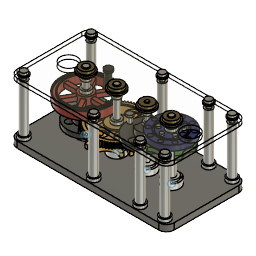
DualStageGenevaIndexingMechanism_2_5D_AI_Model (Autodesk Fusion 360 design; units mm, degrees)
part number: 2026-08-16-05-34-55-239
part number: 2026-08-16-05-35-11-169
part number: 2026-08-16-05-35-42-913
part number: 2026-08-16-05-35-42-976
part number: 2026-08-16-05-35-43-045
part number: 2026-08-16-05-35-43-120
part number: 2026-08-16-05-35-43-201
part number: 2026-08-16-05-36-34-609
part number: 2026-08-16-05-36-34-765
part number: 2026-08-16-05-36-34-899
part number: 2026-08-16-05-36-35-022
part number: 2026-08-16-05-37-12-410
part number: 2026-08-16-05-37-12-675
part number: 2026-08-16-05-39-24-332
part number: 2026-08-16-05-39-24-566
part number: 2026-08-16-05-40-07-479
part number: 2026-08-16-05-41-21-230
part number: 2026-08-16-05-43-01-261
part number: 2026-08-16-05-43-01-779
part number: 2026-08-16-05-43-02-149
part number: 2026-08-16-05-44-14-801
part number: 2026-08-16-05-44-15-447
part number: 2026-08-16-05-45-26-077
part number: 2026-08-16-05-45-26-591
part number: 2026-08-16-05-45-26-921
part number: 2026-08-16-05-45-27-444
Autodesk Fusion 360 part; units mm, degrees
note: some values were not read from the file. Chosen so that the rebuilt part matches the saved one: which bodies a step acts on. Set by a fixed rule: which sketch regions a step uses.
(part 1 of 6)
sketch "スケッチ1" plane through (0, 0, 0) normal (0, 0, 1) x (1, 0, 0) in component "Lower_Base_Plate"
  line L0 (-290, -125) -> (200, -125)
  line L1 (200, -125) -> (200, 125)
  line L2 (200, 125) -> (-290, 125)
  line L3 (-290, 125) -> (-290, -125)
extrude "押し出し1" add sketch "スケッチ1" along normal blind 20 from surface at -20 makes body 1 in component "Lower_Base_Plate"
fillet "フィレット1" radius 24 4 edges at (-290, 125, -10) (200, 125, -10) (200, -125, -10) (-290, -125, -10) on bodies 1 in component "Lower_Base_Plate"
sketch "スケッチ1 (2)" plane through (0, 0, 0) normal (0, 0, 1) x (1, 0, 0) in component "Bearing_Housing_A"
  circle A0 centre (-176, 0) radius 26
extrude "押し出し1'" add sketch "スケッチ1 (2)" along normal blind 18 separate body makes body 2 in component "Bearing_Housing_A"
sketch "スケッチ2" plane through (0, 0, 0) normal (0, 0, 1) x (1, 0, 0) in component "Bearing_Housing_A"
  circle A0 centre (-176, 0) radius 20
extrude "押し出し2" add sketch "スケッチ2" along normal blind 6 from surface at 18 bodies 2 in component "Bearing_Housing_A"
sketch "スケッチ3" plane through (0, 0, 0) normal (0, 0, 1) x (1, 0, 0) in component "Bearing_Housing_A"
  circle A0 centre (-176, 0) radius 10
  circle A1 centre (-160.0901, 15.9099) radius 3
  circle A2 centre (-191.9099, 15.9099) radius 3
  circle A3 centre (-191.9099, -15.9099) radius 3
  circle A4 centre (-160.0901, -15.9099) radius 3
extrude "押し出し3" cut sketch "スケッチ3" along normal blind 40 from surface at -5 bodies 2 in component "Bearing_Housing_A"
sketch "スケッチ1 (3)" plane through (0, 0, 0) normal (0, 0, 1) x (1, 0, 0) in component "Bearing_Housing_B"
  circle A0 centre (-80, 0) radius 26
extrude "押し出し1''" add sketch "スケッチ1 (3)" along normal blind 18 separate body makes body 3 in component "Bearing_Housing_B"
sketch "スケッチ2 (2)" plane through (0, 0, 0) normal (0, 0, 1) x (1, 0, 0) in component "Bearing_Housing_B"
  circle A0 centre (-80, 0) radius 20
extrude "押し出し2'" add sketch "スケッチ2 (2)" along normal blind 6 from surface at 18 bodies 3 in component "Bearing_Housing_B"
sketch "スケッチ3 (2)" plane through (0, 0, 0) normal (0, 0, 1) x (1, 0, 0) in component "Bearing_Housing_B"
  circle A0 centre (-80, 0) radius 9
  circle A1 centre (-64.0901, 15.9099) radius 3
  circle A2 centre (-95.9099, 15.9099) radius 3
  circle A3 centre (-95.9099, -15.9099) radius 3
  circle A4 centre (-64.0901, -15.9099) radius 3
extrude "押し出し3'" cut sketch "スケッチ3 (2)" along normal blind 40 from surface at -5 bodies 3 in component "Bearing_Housing_B"
sketch "スケッチ1 (4)" plane through (0, 0, 0) normal (0, 0, 1) x (1, 0, 0) in component "Bearing_Housing_C"
  circle A0 centre (14.5, 0) radius 26
extrude "押し出し1'''" add sketch "スケッチ1 (4)" along normal blind 18 separate body makes body 4 in component "Bearing_Housing_C"
sketch "スケッチ2 (3)" plane through (0, 0, 0) normal (0, 0, 1) x (1, 0, 0) in component "Bearing_Housing_C"
  circle A0 centre (14.5, 0) radius 20
extrude "押し出し2''" add sketch "スケッチ2 (3)" along normal blind 6 from surface at 18 bodies 4 in component "Bearing_Housing_C"
sketch "スケッチ3 (3)" plane through (0, 0, 0) normal (0, 0, 1) x (1, 0, 0) in component "Bearing_Housing_C"
  circle A0 centre (14.5, 0) radius 6
  circle A1 centre (30.4099, 15.9099) radius 3
  circle A2 centre (-1.4099, 15.9099) radius 3
  circle A3 centre (-1.4099, -15.9099) radius 3
  circle A4 centre (30.4099, -15.9099) radius 3
extrude "押し出し3''" cut sketch "スケッチ3 (3)" along normal blind 40 from surface at -5 bodies 4 in component "Bearing_Housing_C"
sketch "スケッチ1 (5)" plane through (0, 0, 0) normal (0, 0, 1) x (1, 0, 0) in component "Bearing_Housing_D"
  circle A0 centre (90.5, 0) radius 26
extrude "押し出し1''''" add sketch "スケッチ1 (5)" along normal blind 18 separate body makes body 5 in component "Bearing_Housing_D"
sketch "スケッチ2 (4)" plane through (0, 0, 0) normal (0, 0, 1) x (1, 0, 0) in component "Bearing_Housing_D"
  circle A0 centre (90.5, 0) radius 20
extrude "押し出し2'''" add sketch "スケッチ2 (4)" along normal blind 6 from surface at 18 bodies 5 in component "Bearing_Housing_D"
sketch "スケッチ3 (4)" plane through (0, 0, 0) normal (0, 0, 1) x (1, 0, 0) in component "Bearing_Housing_D"
  circle A0 centre (90.5, 0) radius 9
  circle A1 centre (106.4099, 15.9099) radius 3
  circle A2 centre (74.5901, 15.9099) radius 3
  circle A3 centre (74.5901, -15.9099) radius 3
  circle A4 centre (106.4099, -15.9099) radius 3
extrude "押し出し3'''" cut sketch "スケッチ3 (4)" along normal blind 40 from surface at -5 bodies 5 in component "Bearing_Housing_D"
sketch "スケッチ1 (6)" plane through (0, 0, 0) normal (0, 0, 1) x (1, 0, 0) in component "Standoff_Posts"
  circle A0 centre (-265, 105) radius 12
  circle A1 centre (-265, -105) radius 12
  circle A2 centre (-45, 107) radius 12
  circle A3 centre (-45, -107) radius 12
  circle A4 centre (100, 107) radius 12
  circle A5 centre (100, -107) radius 12
  circle A6 centre (175, 105) radius 12
  circle A7 centre (175, -105) radius 12
extrude "押し出し1'''''" add sketch "スケッチ1 (6)" along normal blind 158 separate body makes body 6 at (186.9404, 103.8052, 105.3333) makes body 7 at (111.9404, 105.8052, 105.3333) makes body 8 at (-33.0596, -108.1948, 105.3333) makes body 9 at (-270.4745, -115.6785, 52.6667) makes body 10 at (-33.0596, 105.8052, 105.3333) makes body 11 at (-270.4745, 94.3215, 52.6667) makes body 12 at (111.9404, -108.1948, 105.3333) makes body 13 at (186.9404, -106.1948, 105.3333) in component "Standoff_Posts"
sketch "スケッチ2 (5)" plane through (0, 0, 0) normal (0, 0, 1) x (1, 0, 0) in component "Standoff_Posts"
  circle A0 centre (-265, 105) radius 16
  circle A1 centre (-265, -105) radius 16
  circle A2 centre (-45, 107) radius 16
  circle A3 centre (-45, -107) radius 16
  circle A4 centre (100, 107) radius 16
  circle A5 centre (100, -107) radius 16
  circle A6 centre (175, 105) radius 16
  circle A7 centre (175, -105) radius 16
extrude "押し出し2''''" add sketch "スケッチ2 (5)" along normal blind 10 bodies 6 7 8 9 10 11 12 13 in component "Standoff_Posts"
sketch "スケッチ3 (5)" plane through (0, 0, 0) normal (0, 0, 1) x (1, 0, 0) in component "Standoff_Posts"
  circle A0 centre (-265, 105) radius 6
  circle A1 centre (-265, -105) radius 6
  circle A2 centre (-45, 107) radius 6
  circle A3 centre (-45, -107) radius 6
  circle A4 centre (100, 107) radius 6
  circle A5 centre (100, -107) radius 6
  circle A6 centre (175, 105) radius 6
  circle A7 centre (175, -105) radius 6
extrude "押し出し3''''" cut sketch "スケッチ3 (5)" along normal blind 20 from surface at 140 bodies 6 7 8 9 10 11 12 13 in component "Standoff_Posts"
sketch "スケッチ1 (7)" plane through (0, 0, 0) normal (0, 0, 1) x (1, 0, 0) in component "Input_Shaft"
  circle A0 centre (-176, 0) radius 9
extrude "押し出し1''''''" add sketch "スケッチ1 (7)" along normal blind 186 separate body makes body 14 in component "Input_Shaft"
sketch "スケッチ2 (6)" plane through (0, 0, 0) normal (0, 0, 1) x (1, 0, 0) in component "Input_Shaft"
  circle A0 centre (-176, 0) radius 14
extrude "押し出し2'''''" add sketch "スケッチ2 (6)" along normal blind 4 from surface at 24 bodies 14 in component "Input_Shaft"
sketch "スケッチ3 (6)" plane through (0, 0, 0) normal (0, 0, 1) x (1, 0, 0) in component "Input_Shaft"
  circle A0 centre (-176, 0) radius 10
extrude "押し出し3'''''" add sketch "スケッチ3 (6)" along normal blind 20 from surface at 62 bodies 14 in component "Input_Shaft"
sketch "スケッチ4" plane through (0, 0, 0) normal (0, 0, 1) x (1, 0, 0) in component "Input_Shaft"
  circle A0 centre (-176, 0) radius 11
extrude "押し出し4" add sketch "スケッチ4" along normal blind 10 from surface at 82 bodies 14 in component "Input_Shaft"
sketch "スケッチ5" plane through (0, 0, 0) normal (0, 0, 1) x (1, 0, 0) in component "Input_Shaft"
  circle A0 centre (-176, 0) radius 15
extrude "押し出し5" add sketch "スケッチ5" along normal blind 10 from surface at 117 bodies 14 in component "Input_Shaft"
sketch "スケッチ6" plane through (0, 0, 0) normal (0, 0, 1) x (1, 0, 0) in component "Input_Shaft"
  circle A0 centre (-176, 0) radius 13
extrude "押し出し6" add sketch "スケッチ6" along normal blind 8 from surface at 150 bodies 14 in component "Input_Shaft"
sketch "スケッチ7" plane through (0, 0, 0) normal (0, 0, 1) x (1, 0, 0) in component "Input_Shaft"
  circle A0 centre (-176, 0) radius 10.8
sketch "スケッチ1 (8)" plane through (0, 0, 0) normal (0, 0, 1) x (1, 0, 0) in component "Stage1_Shaft"
  circle A0 centre (-80, 0) radius 8
extrude "押し出し1'''''''" add sketch "スケッチ1 (8)" along normal blind 186 separate body makes body 15 in component "Stage1_Shaft"
sketch "スケッチ2 (7)" plane through (0, 0, 0) normal (0, 0, 1) x (1, 0, 0) in component "Stage1_Shaft"
  circle A0 centre (-80, 0) radius 14
extrude "押し出し2''''''" add sketch "スケッチ2 (7)" along normal blind 20 from surface at 24 bodies 15 in component "Stage1_Shaft"
sketch "スケッチ3 (7)" plane through (0, 0, 0) normal (0, 0, 1) x (1, 0, 0) in component "Stage1_Shaft"
  circle A0 centre (-80, 0) radius 14
extrude "押し出し3''''''" add sketch "スケッチ3 (7)" along normal blind 6 from surface at 60 bodies 15 in component "Stage1_Shaft"
sketch "スケッチ4 (2)" plane through (0, 0, 0) normal (0, 0, 1) x (1, 0, 0) in component "Stage1_Shaft"
  circle A0 centre (-80, 0) radius 15
extrude "押し出し4'" add sketch "スケッチ4 (2)" along normal blind 10 from surface at 82 bodies 15 in component "Stage1_Shaft"
sketch "スケッチ5 (2)" plane through (0, 0, 0) normal (0, 0, 1) x (1, 0, 0) in component "Stage1_Shaft"
  circle A0 centre (-80, 0) radius 12
extrude "押し出し5'" add sketch "スケッチ5 (2)" along normal blind 8 from surface at 150 bodies 15 in component "Stage1_Shaft"
sketch "スケッチ6 (2)" plane through (0, 0, 0) normal (0, 0, 1) x (1, 0, 0) in component "Stage1_Shaft"
  circle A0 centre (-80, 0) radius 9.8
sketch "スケッチ1 (9)" plane through (0, 0, 0) normal (0, 0, 1) x (1, 0, 0) in component "Stage2_Driver_Shaft"
  circle A0 centre (14.5, 0) radius 5
extrude "押し出し1''''''''" add sketch "スケッチ1 (9)" along normal blind 186 separate body makes body 16 in component "Stage2_Driver_Shaft"
sketch "スケッチ2 (8)" plane through (0, 0, 0) normal (0, 0, 1) x (1, 0, 0) in component "Stage2_Driver_Shaft"
  circle A0 centre (14.5, 0) radius 7
extrude "押し出し2'''''''" add sketch "スケッチ2 (8)" along normal blind 42 from surface at 24 bodies 16 in component "Stage2_Driver_Shaft"
sketch "スケッチ3 (8)" plane through (0, 0, 0) normal (0, 0, 1) x (1, 0, 0) in component "Stage2_Driver_Shaft"
  circle A0 centre (14.5, 0) radius 11
extrude "押し出し3'''''''" add sketch "スケッチ3 (8)" along normal blind 10 from surface at 122 bodies 16 in component "Stage2_Driver_Shaft"
sketch "スケッチ4 (3)" plane through (0, 0, 0) normal (0, 0, 1) x (1, 0, 0) in component "Stage2_Driver_Shaft"
  circle A0 centre (14.5, 0) radius 9
extrude "押し出し4''" add sketch "スケッチ4 (3)" along normal blind 8 from surface at 150 bodies 16 in component "Stage2_Driver_Shaft"
sketch "スケッチ5 (3)" plane through (0, 0, 0) normal (0, 0, 1) x (1, 0, 0) in component "Stage2_Driver_Shaft"
  circle A0 centre (14.5, 0) radius 6.8
sketch "スケッチ1 (10)" plane through (0, 0, 0) normal (0, 0, 1) x (1, 0, 0) in component "Output_Shaft"
  circle A0 centre (90.5, 0) radius 8
extrude "押し出し1'''''''''" add sketch "スケッチ1 (10)" along normal blind 186 separate body makes body 17 in component "Output_Shaft"
sketch "スケッチ2 (9)" plane through (0, 0, 0) normal (0, 0, 1) x (1, 0, 0) in component "Output_Shaft"
  circle A0 centre (90.5, 0) radius 12
extrude "押し出し2''''''''" add sketch "スケッチ2 (9)" along normal blind 76 from surface at 24 bodies 17 in component "Output_Shaft"
sketch "スケッチ3 (9)" plane through (0, 0, 0) normal (0, 0, 1) x (1, 0, 0) in component "Output_Shaft"
  circle A0 centre (90.5, 0) radius 15
extrude "押し出し3''''''''" add sketch "スケッチ3 (9)" along normal blind 10 from surface at 148 bodies 17 in component "Output_Shaft"
sketch "スケッチ4 (4)" plane through (0, 0, 0) normal (0, 0, 1) x (1, 0, 0) in component "Output_Shaft"
  circle A0 centre (90.5, 0) radius 11.15
sketch "スケッチ1 (11)" plane through (0, 0, 0) normal (0, 0, 1) x (1, 0, 0) in component "Input_Handwheel"
  circle A0 centre (-176, 0) radius 78
  circle A1 centre (-176, 0) radius 64
extrude "押し出し1''''''''''" add sketch "スケッチ1 (11)" along normal blind 25 from surface at 92 separate body makes body 18 in component "Input_Handwheel"
sketch "スケッチ2 (10)" plane through (0, 0, 0) normal (0, 0, 1) x (1, 0, 0) in component "Input_Handwheel"
  circle A0 centre (-176, 0) radius 22
  circle A1 centre (-176, 0) radius 9
extrude "押し出し2'''''''''" add sketch "スケッチ2 (10)" along normal blind 25 from surface at 92 bodies 18 makes body 19 in component "Input_Handwheel"
sketch "スケッチ3 (10)" plane through (0, 0, 0) normal (0, 0, 1) x (1, 0, 0) in component "Input_Handwheel"
  line L0 (-160, 6) -> (-110, 6)
  line L1 (-110, 6) -> (-110, -6)
  line L2 (-110, -6) -> (-160, -6)
  line L3 (-160, -6) -> (-160, 6)
  line L4 (-173.1962, 16.8564) -> (-148.1962, 60.1577)
  line L5 (-148.1962, 60.1577) -> (-137.8038, 54.1577)
  line L6 (-137.8038, 54.1577) -> (-162.8038, 10.8564)
  line L7 (-162.8038, 10.8564) -> (-173.1962, 16.8564)
  line L8 (-189.1962, 10.8564) -> (-214.1962, 54.1577)
  line L9 (-214.1962, 54.1577) -> (-203.8038, 60.1577)
  line L10 (-203.8038, 60.1577) -> (-178.8038, 16.8564)
  line L11 (-178.8038, 16.8564) -> (-189.1962, 10.8564)
  line L12 (-192, -6) -> (-242, -6)
  line L13 (-242, -6) -> (-242, 6)
  line L14 (-242, 6) -> (-192, 6)
  line L15 (-192, 6) -> (-192, -6)
  line L16 (-178.8038, -16.8564) -> (-203.8038, -60.1577)
  line L17 (-203.8038, -60.1577) -> (-214.1962, -54.1577)
  line L18 (-214.1962, -54.1577) -> (-189.1962, -10.8564)
  line L19 (-189.1962, -10.8564) -> (-178.8038, -16.8564)
  line L20 (-162.8038, -10.8564) -> (-137.8038, -54.1577)
  line L21 (-137.8038, -54.1577) -> (-148.1962, -60.1577)
  line L22 (-148.1962, -60.1577) -> (-173.1962, -16.8564)
  line L23 (-173.1962, -16.8564) -> (-162.8038, -10.8564)
extrude "押し出し3'''''''''" add sketch "スケッチ3 (10)" along normal blind 13 from surface at 98 bodies 18 in component "Input_Handwheel"
sketch "スケッチ4 (5)" plane through (0, 0, 0) normal (0, 0, 1) x (1, 0, 0) in component "Input_Handwheel"
  circle A0 centre (-176, 0) radius 75
  circle A1 centre (-176, 0) radius 67
extrude "押し出し4'''" cut sketch "スケッチ4 (5)" along normal blind 5 from surface at 113 bodies 18 in component "Input_Handwheel"
sketch "スケッチ1 (12)" plane through (0, 0, 0) normal (0, 0, 1) x (1, 0, 0) in component "Input_Crank_Handle"
  circle A0 centre (-176, 70) radius 9
extrude "押し出し1'''''''''''" add sketch "スケッチ1 (12)" along normal blind 32 from surface at 106 separate body makes body 20 in component "Input_Crank_Handle"
sketch "スケッチ2 (11)" plane through (0, 0, 0) normal (0, 0, 1) x (1, 0, 0) in component "Input_Crank_Handle"
  circle A0 centre (-176, 70) radius 12
extrude "押し出し2''''''''''" add sketch "スケッチ2 (11)" along normal blind 6 from surface at 138 bodies 20 in component "Input_Crank_Handle"
sketch "スケッチ5 (4)" plane through (0, 0, 0) normal (0, 0, 1) x (1, 0, 0) in component "Input_Handwheel"
  circle A0 centre (-176, 70) radius 9.4
extrude "押し出し5''" cut sketch "スケッチ5 (4)" along normal blind 36 from surface at 86 bodies 18 in component "Input_Handwheel"
sketch "スケッチ3 (11)" plane through (0, 0, 0) normal (0, 0, 1) x (1, 0, 0) in component "Input_Crank_Handle"
  circle A0 centre (-176, 70) radius 9
extrude "押し出し3''''''''''" add sketch "スケッチ3 (11)" along normal blind 14 from surface at 92 bodies 20 in component "Input_Crank_Handle"
sketch "スケッチ4 (6)" plane through (0, 0, 0) normal (0, 0, 1) x (1, 0, 0) in component "Input_Crank_Handle"
  circle A0 centre (-176, 70) radius 13
extrude "押し出し4''''" add sketch "スケッチ4 (6)" along normal blind 8 from surface at 84 bodies 20 in component "Input_Crank_Handle"
combine "結合1" operation add target body 18 tool bodies 19 in component "Input_Handwheel"
sketch "スケッチ1 (13)" plane through (0, 0, 0) normal (0, 0, 1) x (1, 0, 0) in component "Stage1_Driver_Disc"
  circle A0 centre (-176, 0) radius 58
extrude "押し出し1''''''''''''" add sketch "スケッチ1 (13)" along normal blind 14 from surface at 28 separate body makes body 21 in component "Stage1_Driver_Disc"
sketch "スケッチ2 (12)" plane through (0, 0, 0) normal (0, 0, 1) x (1, 0, 0) in component "Stage1_Driver_Disc"
  circle A0 centre (-176, 0) radius 16
extrude "押し出し2'''''''''''" add sketch "スケッチ2 (12)" along normal blind 34 from surface at 28 bodies 21 in component "Stage1_Driver_Disc"
sketch "スケッチ3 (12)" plane through (0, 0, 0) normal (0, 0, 1) x (1, 0, 0) in component "Stage1_Driver_Disc"
  circle A0 centre (-176, 0) radius 32
  circle A1 centre (-128, 83.1384) radius 86
extrude "押し出し3'''''''''''" add sketch "スケッチ3 (12)" along normal blind 20 from surface at 42 contours A0 A1 picked at (-177.9353, -3.352) bodies 21 in component "Stage1_Driver_Disc"
sketch "スケッチ4 (7)" plane through (0, 0, 0) normal (0, 0, 1) x (1, 0, 0) in component "Stage1_Driver_Disc"
  circle A0 centre (-208.909, 19) radius 11
  circle A1 centre (-195, -32.909) radius 11
  circle A2 centre (-143.091, -19) radius 11
extrude "押し出し4'''''" cut sketch "スケッチ4 (7)" along normal blind 14 from surface at 28 bodies 21 in component "Stage1_Driver_Disc"
sketch "スケッチ5 (5)" plane through (0, 0, 0) normal (0, 0, 1) x (1, 0, 0) in component "Stage1_Driver_Disc"
  circle A0 centre (-176, 0) radius 9
extrude "押し出し5'''" cut sketch "スケッチ5 (5)" along normal blind 42 from surface at 24 bodies 21 in component "Stage1_Driver_Disc"
sketch "スケッチ1 (14)" plane through (0, 0, 0) normal (0, 0, 1) x (1, 0, 0) in component "Stage1_Drive_Pin"
  circle A0 centre (-152, 41.5692) radius 6
extrude "押し出し1'''''''''''''" add sketch "スケッチ1 (14)" along normal blind 22 from surface at 42 separate body makes body 22 in component "Stage1_Drive_Pin"
sketch "スケッチ2 (13)" plane through (0, 0, 0) normal (0, 0, 1) x (1, 0, 0) in component "Stage1_Drive_Pin"
  circle A0 centre (-152, 41.5692) radius 9.5
extrude "押し出し2''''''''''''" add sketch "スケッチ2 (13)" along normal blind 6 from surface at 58 bodies 22 in component "Stage1_Drive_Pin"
sketch "スケッチ1 (15)" plane through (0, 0, 0) normal (0, 0, 1) x (1, 0, 0) in component "Stage1_Geneva_Wheel_6Slot"
  circle A0 centre (-80, 0) radius 85
extrude "押し出し1''''''''''''''" add sketch "スケッチ1 (15)" along normal blind 12 from surface at 46 separate body makes body 23 in component "Stage1_Geneva_Wheel_6Slot"
sketch "スケッチ2 (14)" plane through (0, 0, 0) normal (0, 0, 1) x (1, 0, 0) in component "Stage1_Geneva_Wheel_6Slot"
  circle A0 centre (-80, 0) radius 22
extrude "押し出し2'''''''''''''" add sketch "スケッチ2 (14)" along normal blind 16 from surface at 44 bodies 23 in component "Stage1_Geneva_Wheel_6Slot"
sketch "スケッチ3 (13)" plane through (0, 0, 0) normal (0, 0, 1) x (1, 0, 0) in component "Stage1_Geneva_Wheel_6Slot"
  line L0 (-124.8192, 18.3708) -> (-163.7904, 40.8708)
  line L1 (-163.7904, 40.8708) -> (-157.2904, 52.1292)
  line L2 (-157.2904, 52.1292) -> (-118.3192, 29.6292)
  arc A0 (-124.8192, 18.3708) -> (-118.3192, 29.6292) centre (-121.5692, 24) ccw
  line L3 (-118.3192, -29.6292) -> (-157.2904, -52.1292)
  line L4 (-157.2904, -52.1292) -> (-163.7904, -40.8708)
  line L5 (-163.7904, -40.8708) -> (-124.8192, -18.3708)
  arc A1 (-118.3192, -29.6292) -> (-124.8192, -18.3708) centre (-121.5692, -24) ccw
  line L6 (-73.5, -48) -> (-73.5, -93)
  line L7 (-73.5, -93) -> (-86.5, -93)
  line L8 (-86.5, -93) -> (-86.5, -48)
  arc A2 (-73.5, -48) -> (-86.5, -48) centre (-80, -48) ccw
  line L9 (-35.1808, -18.3708) -> (3.7904, -40.8708)
  line L10 (3.7904, -40.8708) -> (-2.7096, -52.1292)
  line L11 (-2.7096, -52.1292) -> (-41.6808, -29.6292)
  arc A3 (-35.1808, -18.3708) -> (-41.6808, -29.6292) centre (-38.4308, -24) ccw
  line L12 (-41.6808, 29.6292) -> (-2.7096, 52.1292)
  line L13 (-2.7096, 52.1292) -> (3.7904, 40.8708)
  line L14 (3.7904, 40.8708) -> (-35.1808, 18.3708)
  arc A4 (-41.6808, 29.6292) -> (-35.1808, 18.3708) centre (-38.4308, 24) ccw
  line L15 (-86.5, 48) -> (-86.5, 93)
  line L16 (-86.5, 93) -> (-73.5, 93)
  line L17 (-73.5, 93) -> (-73.5, 48)
  arc A5 (-86.5, 48) -> (-73.5, 48) centre (-80, 48) ccw
extrude "押し出し3''''''''''''" cut sketch "スケッチ3 (13)" along normal blind 20 from surface at 42 bodies 23 in component "Stage1_Geneva_Wheel_6Slot"
sketch "スケッチ4 (8)" plane through (0, 0, 0) normal (0, 0, 1) x (1, 0, 0) in component "Stage1_Geneva_Wheel_6Slot"
  circle A0 centre (-176, 0) radius 32
  circle A1 centre (-128, -83.1384) radius 32
  circle A2 centre (-32, -83.1384) radius 32
  circle A3 centre (16, 0) radius 32
  circle A4 centre (-32, 83.1384) radius 32
  circle A5 centre (-128, 83.1384) radius 32
extrude "押し出し4''''''" cut sketch "スケッチ4 (8)" along normal blind 20 from surface at 42 bodies 23 in component "Stage1_Geneva_Wheel_6Slot"
sketch "スケッチ5 (6)" plane through (0, 0, 0) normal (0, 0, 1) x (1, 0, 0) in component "Stage1_Geneva_Wheel_6Slot"
  circle A0 centre (-122, 0) radius 11
  circle A1 centre (-101, -36.3731) radius 11
  circle A2 centre (-59, -36.3731) radius 11
  circle A3 centre (-38, 0) radius 11
  circle A4 centre (-59, 36.3731) radius 11
  circle A5 centre (-101, 36.3731) radius 11
extrude "押し出し5''''" cut sketch "スケッチ5 (6)" along normal blind 20 from surface at 42 bodies 23 in component "Stage1_Geneva_Wheel_6Slot"
sketch "スケッチ6 (3)" plane through (0, 0, 0) normal (0, 0, 1) x (1, 0, 0) in component "Stage1_Geneva_Wheel_6Slot"
  circle A0 centre (-80, 0) radius 8
extrude "押し出し6'" cut sketch "スケッチ6 (3)" along normal blind 24 from surface at 40 bodies 23 in component "Stage1_Geneva_Wheel_6Slot"
sketch "スケッチ1 (16)" plane through (0, 0, 0) normal (0, 0, 1) x (1, 0, 0) in component "Intermediate_Spur_Gear_72T"
  spline S0 degree 5 poles (3.2013, 2.8471) (3.1556, 2.825) (3.0643, 2.7811) (2.9279, 2.7161) (2.7471, 2.631) (2.5228, 2.5275) (2.3003, 2.4268) (2.0797, 2.329) (1.8609, 2.2341) (1.644, 2.1421) (1.4292, 2.0529) (1.2166, 1.9667) (1.0061, 1.8834) (0.798, 1.8029) (0.5923, 1.7252) (0.389, 1.6503) (0.1883, 1.5783) (-0.0098, 1.5091) (-0.2052, 1.4426) (-0.3978, 1.379) (-0.5873, 1.3182) (-0.7737, 1.2602) (-0.9567, 1.2049) (-1.1363, 1.1524) (-1.3124, 1.1026) (-1.4849, 1.0555) (-1.6201, 1.02) (-1.7199, 0.9945) (-1.7858, 0.9781) (-1.8185, 0.97) knots 0 0 0 0 0 0 0.04 0.08 0.12 0.16 0.2 0.24 0.28 0.32 0.36 0.4 0.44 0.48 0.52 0.56 0.6 0.64 0.68 0.72 0.76 0.8 0.84 0.88 0.92 0.96 1 1 1 1 1 1
  arc A0 (-1.8185, 0.97) -> (3.1328, 4.4152) centre (-0.1573, 3.8631) ccw
  spline S1 degree 5 poles (3.1328, 4.4152) (3.0854, 4.4332) (2.9906, 4.469) (2.8491, 4.5219) (2.6616, 4.5909) (2.4291, 4.6744) (2.1987, 4.7554) (1.9703, 4.8336) (1.7441, 4.9091) (1.52, 4.9818) (1.2983, 5.0519) (1.0789, 5.1193) (0.862, 5.184) (0.6477, 5.246) (0.436, 5.3055) (0.227, 5.3623) (0.0207, 5.4166) (-0.1827, 5.4683) (-0.3831, 5.5174) (-0.5805, 5.564) (-0.7746, 5.6081) (-0.9653, 5.6497) (-1.1525, 5.6888) (-1.336, 5.7254) (-1.5157, 5.7596) (-1.6917, 5.7915) (-1.8295, 5.8151) (-1.9311, 5.8318) (-1.9982, 5.8425) (-2.0315, 5.8477) knots 0 0 0 0 0 0 0.04 0.08 0.12 0.16 0.2 0.24 0.28 0.32 0.36 0.4 0.44 0.48 0.52 0.56 0.6 0.64 0.68 0.72 0.76 0.8 0.84 0.88 0.92 0.96 1 1 1 1 1 1
  arc A1 (2.6366, 10.0878) -> (-2.0315, 5.8477) centre (1.5239, 6.6231) ccw
  spline S2 degree 5 poles (2.6366, 10.0878) (2.5929, 10.0618) (2.5058, 10.0101) (2.3757, 9.9334) (2.2029, 9.8329) (1.9885, 9.7102) (1.7757, 9.5905) (1.5643, 9.4739) (1.3546, 9.3602) (1.1466, 9.2496) (0.9404, 9.1422) (0.7361, 9.0377) (0.5337, 8.9363) (0.3334, 8.838) (0.1352, 8.7427) (-0.0607, 8.6504) (-0.2544, 8.5612) (-0.4457, 8.4749) (-0.6346, 8.3917) (-0.8209, 8.3116) (-1.0044, 8.2345) (-1.185, 8.1604) (-1.3625, 8.0894) (-1.5369, 8.0214) (-1.7079, 7.9565) (-1.8757, 7.8946) (-2.0073, 7.8474) (-2.1045, 7.8133) (-2.1686, 7.7912) (-2.2006, 7.7802) knots 0 0 0 0 0 0 0.04 0.08 0.12 0.16 0.2 0.24 0.28 0.32 0.36 0.4 0.44 0.48 0.52 0.56 0.6 0.64 0.68 0.72 0.76 0.8 0.84 0.88 0.92 0.96 1 1 1 1 1 1
  arc A2 (-2.2006, 7.7802) -> (2.4317, 11.6439) centre (-0.7979, 10.8072) ccw
  spline S3 degree 5 poles (2.4317, 11.6439) (2.3828, 11.6577) (2.2853, 11.6851) (2.1397, 11.7255) (1.9469, 11.7778) (1.708, 11.8408) (1.4714, 11.9013) (1.2371, 11.9594) (1.0051, 12.0149) (0.7756, 12.0678) (0.5486, 12.1183) (0.3242, 12.1663) (0.1025, 12.2118) (-0.1164, 12.255) (-0.3325, 12.2957) (-0.5457, 12.3341) (-0.7559, 12.3702) (-0.963, 12.404) (-1.1669, 12.4355) (-1.3676, 12.4647) (-1.5649, 12.4917) (-1.7585, 12.5165) (-1.9483, 12.5391) (-2.1343, 12.5596) (-2.3164, 12.5781) (-2.4944, 12.5945) (-2.6337, 12.606) (-2.7365, 12.6138) (-2.8042, 12.6186) (-2.8378, 12.6208) knots 0 0 0 0 0 0 0.04 0.08 0.12 0.16 0.2 0.24 0.28 0.32 0.36 0.4 0.44 0.48 0.52 0.56 0.6 0.64 0.68 0.72 0.76 0.8 0.84 0.88 0.92 0.96 1 1 1 1 1 1
  arc A3 (1.4429, 17.2516) -> (-2.8378, 12.6208) centre (0.6364, 13.7032) ccw
  spline S4 degree 5 poles (1.4429, 17.2516) (1.4017, 17.2219) (1.3194, 17.1628) (1.1964, 17.0751) (1.0331, 16.96) (0.8302, 16.8191) (0.6286, 16.6813) (0.4283, 16.5466) (0.2293, 16.4151) (0.0317, 16.2868) (-0.1644, 16.1618) (-0.3588, 16.0399) (-0.5516, 15.9213) (-0.7426, 15.8059) (-0.9317, 15.6937) (-1.1188, 15.5847) (-1.304, 15.4789) (-1.4871, 15.3763) (-1.668, 15.277) (-1.8466, 15.1809) (-2.0227, 15.088) (-2.1961, 14.9985) (-2.3668, 14.9123) (-2.5345, 14.8294) (-2.6993, 14.7498) (-2.861, 14.6735) (-2.988, 14.615) (-3.0819, 14.5726) (-3.1439, 14.545) (-3.1747, 14.5313) knots 0 0 0 0 0 0 0.04 0.08 0.12 0.16 0.2 0.24 0.28 0.32 0.36 0.4 0.44 0.48 0.52 0.56 0.6 0.64 0.68 0.72 0.76 0.8 0.84 0.88 0.92 0.96 1 1 1 1 1 1
  arc A4 (-3.1747, 14.5313) -> (1.1032, 18.784) centre (-2.0411, 17.669) ccw
  spline S5 degree 5 poles (1.1032, 18.784) (1.0533, 18.7935) (0.9538, 18.8123) (0.8052, 18.8398) (0.6086, 18.8751) (0.3651, 18.9171) (0.1241, 18.9568) (-0.1143, 18.9941) (-0.3503, 19.0292) (-0.5835, 19.062) (-0.8141, 19.0924) (-1.0418, 19.1207) (-1.2666, 19.1467) (-1.4885, 19.1706) (-1.7073, 19.1924) (-1.923, 19.2121) (-2.1356, 19.2297) (-2.3448, 19.2453) (-2.5508, 19.2589) (-2.7532, 19.2705) (-2.952, 19.2802) (-3.1471, 19.2881) (-3.3382, 19.2941) (-3.5253, 19.2983) (-3.7082, 19.3008) (-3.887, 19.3016) (-4.0268, 19.301) (-4.1298, 19.2997) (-4.1977, 19.2986) (-4.2314, 19.2979) knots 0 0 0 0 0 0 0.04 0.08 0.12 0.16 0.2 0.24 0.28 0.32 0.36 0.4 0.44 0.48 0.52 0.56 0.6 0.64 0.68 0.72 0.76 0.8 0.84 0.88 0.92 0.96 1 1 1 1 1 1
  arc A5 (-0.3706, 24.2842) -> (-4.2314, 19.2979) centre (-0.8648, 20.679) ccw
  spline S6 degree 5 poles (-0.3706, 24.2842) (-0.409, 24.251) (-0.4858, 24.185) (-0.6007, 24.0869) (-0.7534, 23.9579) (-0.9432, 23.7999) (-1.1321, 23.645) (-1.3199, 23.4934) (-1.5067, 23.3451) (-1.6923, 23.2001) (-1.8768, 23.0584) (-2.0599, 22.9201) (-2.2416, 22.7851) (-2.4217, 22.6535) (-2.6003, 22.5252) (-2.7773, 22.4003) (-2.9525, 22.2788) (-3.126, 22.1606) (-3.2975, 22.0459) (-3.467, 21.9346) (-3.6344, 21.8268) (-3.7994, 21.7225) (-3.9619, 21.6218) (-4.1218, 21.5246) (-4.279, 21.4309) (-4.4334, 21.3408) (-4.5548, 21.2715) (-4.6447, 21.221) (-4.704, 21.1881) (-4.7335, 21.1718) knots 0 0 0 0 0 0 0.04 0.08 0.12 0.16 0.2 0.24 0.28 0.32 0.36 0.4 0.44 0.48 0.52 0.56 0.6 0.64 0.68 0.72 0.76 0.8 0.84 0.88 0.92 0.96 1 1 1 1 1 1
  arc A6 (-4.7335, 21.1718) -> (-0.8426, 25.7811) centre (-3.8778, 24.3963) ccw
  spline S7 degree 5 poles (-0.8426, 25.7811) (-0.8931, 25.7862) (-0.9939, 25.7963) (-1.1443, 25.8107) (-1.3433, 25.8288) (-1.5894, 25.8494) (-1.833, 25.8679) (-2.0738, 25.8843) (-2.3119, 25.8987) (-2.5471, 25.911) (-2.7794, 25.9213) (-3.0087, 25.9296) (-3.235, 25.9359) (-3.4581, 25.9404) (-3.678, 25.943) (-3.8946, 25.9439) (-4.1078, 25.9429) (-4.3177, 25.9402) (-4.524, 25.9358) (-4.7267, 25.9297) (-4.9256, 25.922) (-5.1206, 25.9128) (-5.3115, 25.9021) (-5.4982, 25.8901) (-5.6807, 25.8766) (-5.8589, 25.8619) (-5.9981, 25.849) (-6.1006, 25.8388) (-6.1681, 25.8318) (-6.2017, 25.8282) knots 0 0 0 0 0 0 0.04 0.08 0.12 0.16 0.2 0.24 0.28 0.32 0.36 0.4 0.44 0.48 0.52 0.56 0.6 0.64 0.68 0.72 0.76 0.8 0.84 0.88 0.92 0.96 1 1 1 1 1 1
  arc A7 (-2.7901, 31.1319) -> (-6.2017, 25.8282) centre (-2.9682, 27.4974) ccw
  spline S8 degree 5 poles (-2.7901, 31.1319) (-2.8255, 31.0955) (-2.8963, 31.0231) (-3.0022, 30.9153) (-3.143, 30.7736) (-3.3184, 30.5996) (-3.493, 30.4288) (-3.6669, 30.2614) (-3.8401, 30.0974) (-4.0124, 29.9368) (-4.1837, 29.7796) (-4.3541, 29.6258) (-4.5233, 29.4755) (-4.6913, 29.3287) (-4.8581, 29.1853) (-5.0235, 29.0455) (-5.1875, 28.9091) (-5.3499, 28.7763) (-5.5108, 28.6471) (-5.67, 28.5214) (-5.8273, 28.3994) (-5.9826, 28.2812) (-6.1357, 28.1666) (-6.2865, 28.0559) (-6.4349, 27.9489) (-6.581, 27.8456) (-6.6958, 27.766) (-6.7809, 27.7079) (-6.8372, 27.6699) (-6.8652, 27.6511) knots 0 0 0 0 0 0 0.04 0.08 0.12 0.16 0.2 0.24 0.28 0.32 0.36 0.4 0.44 0.48 0.52 0.56 0.6 0.64 0.68 0.72 0.76 0.8 0.84 0.88 0.92 0.96 1 1 1 1 1 1
  arc A8 (-6.8652, 27.6511) -> (-3.3908, 32.582) centre (-6.2937, 30.938) ccw
  spline S9 degree 5 poles (-3.3908, 32.582) (-3.4415, 32.5827) (-3.5428, 32.5839) (-3.6939, 32.5852) (-3.8937, 32.5859) (-4.1407, 32.585) (-4.3849, 32.5822) (-4.6263, 32.5776) (-4.8647, 32.5711) (-5.1001, 32.5629) (-5.3325, 32.5529) (-5.5616, 32.5411) (-5.7876, 32.5278) (-6.0102, 32.5128) (-6.2295, 32.4962) (-6.4453, 32.4782) (-6.6577, 32.4586) (-6.8665, 32.4376) (-7.0717, 32.4153) (-7.2731, 32.3915) (-7.4706, 32.3666) (-7.664, 32.3404) (-7.8532, 32.3131) (-8.0382, 32.2848) (-8.2188, 32.2555) (-8.3951, 32.2253) (-8.5326, 32.2003) (-8.6339, 32.1812) (-8.7005, 32.1683) (-8.7336, 32.1618) knots 0 0 0 0 0 0 0.04 0.08 0.12 0.16 0.2 0.24 0.28 0.32 0.36 0.4 0.44 0.48 0.52 0.56 0.6 0.64 0.68 0.72 0.76 0.8 0.84 0.88 0.92 0.96 1 1 1 1 1 1
  arc A9 (-5.7973, 37.7428) -> (-8.7336, 32.1618) centre (-5.6579, 34.1065) ccw
  spline S10 degree 5 poles (-5.7973, 37.7428) (-5.8294, 37.7034) (-5.8935, 37.6251) (-5.9896, 37.5085) (-6.1176, 37.355) (-6.2771, 37.1664) (-6.4362, 36.9811) (-6.5948, 36.7992) (-6.753, 36.6207) (-6.9107, 36.4456) (-7.0677, 36.2741) (-7.224, 36.106) (-7.3795, 35.9416) (-7.5341, 35.7807) (-7.6877, 35.6233) (-7.8403, 35.4696) (-7.9917, 35.3195) (-8.142, 35.173) (-8.291, 35.0302) (-8.4387, 34.8912) (-8.5847, 34.756) (-8.7291, 34.6246) (-8.8717, 34.4971) (-9.0123, 34.3737) (-9.1508, 34.2541) (-9.2873, 34.1386) (-9.3948, 34.0492) (-9.4745, 33.9839) (-9.5272, 33.9412) (-9.5534, 33.92) knots 0 0 0 0 0 0 0.04 0.08 0.12 0.16 0.2 0.24 0.28 0.32 0.36 0.4 0.44 0.48 0.52 0.56 0.6 0.64 0.68 0.72 0.76 0.8 0.84 0.88 0.92 0.96 1 1 1 1 1 1
  arc A10 (-9.5534, 33.92) -> (-6.522, 39.135) centre (-9.2706, 37.2442) ccw
  spline S11 degree 5 poles (-6.522, 39.135) (-6.5726, 39.1312) (-6.6736, 39.1236) (-6.8243, 39.1118) (-7.0234, 39.095) (-7.2694, 39.0725) (-7.5124, 39.0485) (-7.7524, 39.0229) (-7.9894, 38.9957) (-8.2232, 38.9669) (-8.4538, 38.9367) (-8.681, 38.905) (-8.905, 38.872) (-9.1254, 38.8377) (-9.3424, 38.8021) (-9.5559, 38.7653) (-9.7657, 38.7273) (-9.9719, 38.6882) (-10.1744, 38.648) (-10.3729, 38.6069) (-10.5675, 38.5648) (-10.7579, 38.5218) (-10.9441, 38.4782) (-11.1258, 38.4338) (-11.3032, 38.3889) (-11.4762, 38.3434) (-11.611, 38.3066) (-11.7102, 38.2788) (-11.7755, 38.2601) (-11.8079, 38.2507) knots 0 0 0 0 0 0 0.04 0.08 0.12 0.16 0.2 0.24 0.28 0.32 0.36 0.4 0.44 0.48 0.52 0.56 0.6 0.64 0.68 0.72 0.76 0.8 0.84 0.88 0.92 0.96 1 1 1 1 1 1
  arc A11 (-9.3691, 44.0663) -> (-11.8079, 38.2507) centre (-8.9133, 40.4561) ccw
  spline S12 degree 5 poles (-9.3691, 44.0663) (-9.3977, 44.0243) (-9.4548, 43.9407) (-9.5403, 43.8162) (-9.6544, 43.6521) (-9.7969, 43.4503) (-9.9392, 43.2519) (-10.0814, 43.0568) (-10.2235, 42.8652) (-10.3652, 42.6771) (-10.5067, 42.4925) (-10.6478, 42.3115) (-10.7883, 42.1341) (-10.9283, 41.9603) (-11.0676, 41.7902) (-11.2062, 41.6237) (-11.344, 41.461) (-11.481, 41.302) (-11.617, 41.1468) (-11.7519, 40.9954) (-11.8857, 40.8479) (-12.0181, 40.7045) (-12.149, 40.5651) (-12.2783, 40.4299) (-12.4058, 40.2987) (-12.5317, 40.1717) (-12.631, 40.0733) (-12.7047, 40.0013) (-12.7535, 39.9541) (-12.7778, 39.9308) knots 0 0 0 0 0 0 0.04 0.08 0.12 0.16 0.2 0.24 0.28 0.32 0.36 0.4 0.44 0.48 0.52 0.56 0.6 0.64 0.68 0.72 0.76 0.8 0.84 0.88 0.92 0.96 1 1 1 1 1 1
  arc A12 (-12.7778, 39.9308) -> (-10.2124, 45.3901) centre (-12.7858, 43.2669) ccw
  spline S13 degree 5 poles (-10.2124, 45.3901) (-10.2626, 45.3819) (-10.3625, 45.3656) (-10.5115, 45.3406) (-10.7084, 45.3066) (-10.9515, 45.2627) (-11.1915, 45.2176) (-11.4284, 45.1711) (-11.6621, 45.1234) (-11.8925, 45.0744) (-12.1196, 45.0242) (-12.3432, 44.9729) (-12.5634, 44.9204) (-12.7801, 44.867) (-12.9931, 44.8126) (-13.2026, 44.7574) (-13.4083, 44.7013) (-13.6103, 44.6443) (-13.8085, 44.5867) (-14.0027, 44.5283) (-14.1928, 44.4694) (-14.3788, 44.4101) (-14.5604, 44.3504) (-14.7377, 44.2904) (-14.9104, 44.2301) (-15.0788, 44.1698) (-15.2099, 44.1213) (-15.3063, 44.0849) (-15.3697, 44.0607) (-15.4011, 44.0485) knots 0 0 0 0 0 0 0.04 0.08 0.12 0.16 0.2 0.24 0.28 0.32 0.36 0.4 0.44 0.48 0.52 0.56 0.6 0.64 0.68 0.72 0.76 0.8 0.84 0.88 0.92 0.96 1 1 1 1 1 1
  arc A13 (-13.4785, 50.0545) -> (-15.4011, 44.0485) centre (-12.7098, 46.4977) ccw
  spline S14 degree 5 poles (-13.4785, 50.0545) (-13.5033, 50.0102) (-13.5529, 49.9219) (-13.6273, 49.7904) (-13.7266, 49.617) (-13.851, 49.4036) (-13.9755, 49.1935) (-14.1001, 48.9868) (-14.2249, 48.7835) (-14.3498, 48.5838) (-14.4746, 48.3875) (-14.5994, 48.1949) (-14.7239, 48.006) (-14.8482, 47.8206) (-14.9722, 47.639) (-15.0958, 47.4611) (-15.2189, 47.287) (-15.3414, 47.1166) (-15.4634, 46.9502) (-15.5846, 46.7876) (-15.705, 46.6291) (-15.8244, 46.4746) (-15.9426, 46.3244) (-16.0596, 46.1783) (-16.1753, 46.0366) (-16.2896, 45.8991) (-16.38, 45.7924) (-16.4471, 45.7143) (-16.4916, 45.663) (-16.5138, 45.6376) knots 0 0 0 0 0 0 0.04 0.08 0.12 0.16 0.2 0.24 0.28 0.32 0.36 0.4 0.44 0.48 0.52 0.56 0.6 0.64 0.68 0.72 0.76 0.8 0.84 0.88 0.92 0.96 1 1 1 1 1 1
  arc A14 (-16.5138, 45.6376) -> (-14.434, 51.2997) centre (-16.8125, 48.9604) ccw
  spline S15 degree 5 poles (-14.434, 51.2997) (-14.4832, 51.2873) (-14.5814, 51.2622) (-14.7276, 51.2244) (-14.9208, 51.1733) (-15.1592, 51.1085) (-15.3943, 51.0426) (-15.6263, 50.9757) (-15.8549, 50.9077) (-16.0802, 50.8388) (-16.302, 50.769) (-16.5203, 50.6984) (-16.7351, 50.627) (-16.9463, 50.5549) (-17.1538, 50.4821) (-17.3576, 50.4088) (-17.5577, 50.335) (-17.7539, 50.2607) (-17.9463, 50.186) (-18.1347, 50.1109) (-18.319, 50.0357) (-18.4991, 49.9604) (-18.6748, 49.885) (-18.8462, 49.8098) (-19.013, 49.7348) (-19.1755, 49.6599) (-19.3019, 49.6003) (-19.3947, 49.5556) (-19.4557, 49.5259) (-19.486, 49.511) knots 0 0 0 0 0 0 0.04 0.08 0.12 0.16 0.2 0.24 0.28 0.32 0.36 0.4 0.44 0.48 0.52 0.56 0.6 0.64 0.68 0.72 0.76 0.8 0.84 0.88 0.92 0.96 1 1 1 1 1 1
  arc A15 (-18.0942, 55.6618) -> (-19.486, 49.511) centre (-17.0184, 52.1855) ccw
  spline S16 degree 5 poles (-18.0942, 55.6618) (-18.115, 55.6155) (-18.1567, 55.5232) (-18.2194, 55.3857) (-18.3032, 55.2043) (-18.4085, 54.9809) (-18.5142, 54.7607) (-18.6204, 54.5439) (-18.727, 54.3305) (-18.8339, 54.1207) (-18.9412, 53.9143) (-19.0487, 53.7116) (-19.1563, 53.5125) (-19.264, 53.317) (-19.3717, 53.1253) (-19.4793, 52.9373) (-19.5867, 52.7531) (-19.694, 52.5727) (-19.801, 52.3962) (-19.9076, 52.2237) (-20.0137, 52.0553) (-20.1191, 51.891) (-20.2238, 51.7311) (-20.3277, 51.5754) (-20.4305, 51.4241) (-20.5324, 51.2771) (-20.6132, 51.163) (-20.6732, 51.0793) (-20.7131, 51.0244) (-20.733, 50.9971) knots 0 0 0 0 0 0 0.04 0.08 0.12 0.16 0.2 0.24 0.28 0.32 0.36 0.4 0.44 0.48 0.52 0.56 0.6 0.64 0.68 0.72 0.76 0.8 0.84 0.88 0.92 0.96 1 1 1 1 1 1
  arc A16 (-20.733, 50.9971) -> (-19.1546, 56.819) centre (-21.3201, 54.2812) ccw
  spline S17 degree 5 poles (-19.1546, 56.819) (-19.2025, 56.8023) (-19.2981, 56.7688) (-19.4405, 56.7183) (-19.6285, 56.6506) (-19.8603, 56.5652) (-20.0888, 56.4791) (-20.3141, 56.3922) (-20.5359, 56.3046) (-20.7543, 56.2164) (-20.9692, 56.1275) (-21.1805, 56.0381) (-21.3883, 55.9482) (-21.5924, 55.858) (-21.7928, 55.7675) (-21.9894, 55.6767) (-22.1823, 55.5857) (-22.3713, 55.4945) (-22.5564, 55.4033) (-22.7376, 55.3122) (-22.9146, 55.2211) (-23.0875, 55.1304) (-23.256, 55.04) (-23.4201, 54.9502) (-23.5798, 54.8609) (-23.7351, 54.7722) (-23.8558, 54.7017) (-23.9444, 54.6491) (-24.0026, 54.6142) (-24.0315, 54.5968) knots 0 0 0 0 0 0 0.04 0.08 0.12 0.16 0.2 0.24 0.28 0.32 0.36 0.4 0.44 0.48 0.52 0.56 0.6 0.64 0.68 0.72 0.76 0.8 0.84 0.88 0.92 0.96 1 1 1 1 1 1
  arc A17 (-23.181, 60.8454) -> (-24.0315, 54.5968) centre (-21.8064, 57.4761) ccw